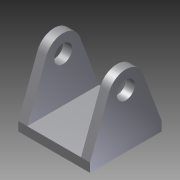
# Autodesk Inventor part: manipulator actuator braket
Saved by Autodesk Inventor 2012 (Build 160160000, 160)
## iProperties
Created: 2013-09-02
Part Number: manipulator actuator braket
Material: Default
Document SubType Name: Modeling
Designer: Bryce
Density: 1 g/cm^3
Author: Bryce
Autodesk Inventor part; units mm, degrees
ref_plane "YZ Plane" through (0, 0, 0) normal (1, 0, 0) x (0, 1, 0)
ref_plane "XZ Plane" through (0, 0, 0) normal (0, 1, 0) x (-1, 0, 0)
ref_plane "XY Plane" through (0, 0, 0) normal (0, 0, 1) x (1, 0, 0)
sketch "Sketch1" plane through (0, 0, 0) normal (0, 0, 1) x (1, 0, 0)
  line L0 (0, 0) -> (25.4, 0)
  line L1 (25.4, 0) -> (25.4, 25.4)
  line L2 (0, 25.4) -> (0, 0)
  line L3 (3.175, 3.175) -> (22.225, 3.175)
  line L4 (22.225, 3.175) -> (22.225, 25.4)
  line L5 (3.175, 25.4) -> (3.175, 3.175)
  line L6 (25.4, 25.4) -> (22.225, 25.4)
  line L7 (3.175, 25.4) -> (0, 25.4)
  dimension "d0" = 25.4
  dimension "d1" = 25.4
  dimension "d2" = 3.175
  dimension "d3" = 3.175
  dimension "d4" = 3.175
  constraints: 16 end point, 4 parallel, 2 horizontal, 2 perpendicular, 1 collinear
  measures "d0" distance of L1.end L2.start
  measures "d1" distance of L2.start L0.start
  measures "d2" distance between parallel lines of L0 L3
  measures "d3" distance between parallel lines of L2 L5
  measures "d4" distance between parallel lines of L1 L4
extrude "Extrusion1" add sketch "Sketch1" along normal blind 25.4
sketch "Sketch2" plane through (25.4, 0, 0) normal (1, 0, 0) x (0, 0, -1)
  line L0 (-25.4, 25.4) -> (-25.4, 0) projected
  line L1 (0, 0) -> (-25.4, 0) projected
  line L2 (0, 0) -> (0, 25.4) projected
  line L3 (0, 25.4) -> (-25.4, 25.4) projected
  arc A0 (-6.7505, 21.2696) -> (-18.6495, 21.2696) centre (-12.7, 19.05) ccw
  circle A1 centre (-12.7, 19.05) radius 3.175
  line L4 (-25.4, 3.175) -> (-18.6495, 21.2696)
  line L5 (0, 3.175) -> (-6.7505, 21.2696)
  dimension "d7" = 19.05
  dimension "d8" = 12.7
  dimension "d9" = 6.35
  dimension "d10" = 3.175
  dimension "d11" = 3.175
  constraints: 4 end point, 3 tangent, 2 centre point, 2 point on circle, 2 point on line, 1 coincident
  measures "d7" distance from line of L1 A0.centre
  measures "d8" distance from line of L0 A0.centre
  measures "d9" diameter of A1
  measures "d10" distance from line of L1 L4.start
  measures "d11" distance of L1.start L5.start
extrude "Extrusion2" cut sketch "Sketch2" against normal blind 25.4 contours L3 A0 L4 L0 | L3 L2 L5 A0 | A1
equation "\"d1\" = d0"
equation "\"d3\" = d2"
equation "\"d4\" = d2"
equation "\"d11\" = d10"
body "Solid1"
